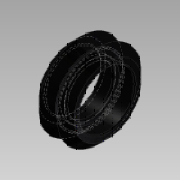
# Autodesk Inventor part: Dual V Wheel
Saved by Autodesk Inventor 2013 SP2 (Build 170200200, 200)
## iProperties
Created: 2013-06-20
Part Number: Dual V Wheel
Material: Acetal Resin, Black
Document SubType Name: Modeling
Designer: Jon Hollander
Language: en-US
Size Designation: Dual V Wheel
Categories: <MemberInstance><Categories><Category DisplayName="Other Parts" InternalName="5aa15e00-363f-49f2-933f-16f664388e3f" Mnemonic="OTHER"><Category DisplayName="Wheel Parts" InternalName="9b824a2a-da77-471e-9ca4-422f1cf2c5b3" Mnemonic="WHEEL PARTS"/></Category><Category DisplayName="DataType" InternalName="23b78d0f-2648-40c6-8793-ca6db495c9e8" Mnemonic="DATATYPE"><CategoryParameter DisplayName="DisplayName" InternalName="05415f3d-3907-474b-a020-eb9d644f4cf3" Mnemonic="DISPLAYNAME"/><CategoryParameter DisplayName="InternalName" InternalName="cf1d0246-76d9-4b4a-8305-fa0409afb5c1" Mnemonic="INTERNALNAME"/><CategoryParameter DisplayName="Folder Name" InternalName="3f06958e-8713-4116-9be7-ed6184ecc97b" Mnemonic="FOLDERNAME"/><CategoryParameter DisplayName="Family Version" InternalName="914462f6-6e19-4b14-ba84-155b9680b1d0" Mnemonic="FAMILYREVISION"/><CategoryParameter DisplayName="ClipFormat" InternalName="bc51e27b-3422-4e78-93ef-cec197ddf230" Mnemonic="CLIPFORMAT"/><CategoryParameter DisplayName="IsMetric" InternalName="e2385c5b-1ea4-4823-96a8-8de651266ec3" Mnemonic="ISMETRIC"/><CategoryParameter DisplayName="Description" InternalName="13903e3d-64b1-4950-80da-f627842ea37f" Mnemonic="DESCRIPTION"/><CategoryParameter DisplayName="StdsOrg" InternalName="8f5914e1-4693-403f-8ab5-d37768198c9d" Mnemonic="STDSORG"/><CategoryParameter DisplayName="Standard" InternalName="0c0a119c-1e12-4c84-803f-101930972f5e" Mnemonic="STANDARD"/><CategoryParameter DisplayName="Manufacturer" InternalName="cd6c7a72-a28a-4e50-99a9-2c7f4e13e5ad" Mnemonic="MANUFACTURER"/><CategoryParameter DisplayName="Member Revision" InternalName="a65d44b9-392f-4f4f-857b-e4b3d54996fe" Mnemonic="MEMBERREVISION"/><CategoryParameter DisplayName="Standard Revision" InternalName="91d5a463-65c2-4fde-b823-3b7fea5e8e17" Mnemonic="STANDARDREVISION"/><CategoryParameter DisplayName="Revision Guid" InternalName="45a75005-10b1-4dfc-8d6d-dfe629f0b93c" Mnemonic="REVISIONGUID"/><CategoryParameter DisplayName="Designation" InternalName="2675968c-4ce5-49e0-a4f5-552d29089031" Mnemonic="DESIGNATION"/><CategoryParameter DisplayName="FileName" InternalName="8b46a4cc-9585-4fed-90c3-899f57e09a73" Mnemonic="FILENAME"/><CategoryParameter DisplayName="Default Row" InternalName="2af9ec52-faaa-4026-b378-f9fa4afca842" Mnemonic="DEFAULTROW"/><Category DisplayName="Part" InternalName="c0e0b642-3bcb-4cc8-9e80-f96d35c4afa4" Mnemonic="PART"><CategoryParameter DisplayName="Material" InternalName="818a152a-d3c3-49ca-80ee-df7d91421b8e" Mnemonic="MATERIAL"/><CategoryParameter DisplayName="Material Key" InternalName="5c9a8adb-dd2b-4535-b97f-0a94a95fe41f" Mnemonic="MATERIALKEY"/><CategoryParameter DisplayName="Part Number" InternalName="016b6077-bfbe-49bd-92c9-d8d59c39c941" Mnemonic="PARTNUMBER"/><CategoryParameter DisplayName="Stock Number" InternalName="4dba7c1c-e26c-444e-836c-b08b433409a8" Mnemonic="STOCKNUMBER"/></Category></Category></Categories><FamilyTemplate Id="Dual V Wheel"><FamilyTemplateParameters><FamilyTemplateParameter ObjectType="kPartComponentDefinitionObject" ValueType="xs:string" Id="11" SubObjectId="Material"/><FamilyTemplateParameter ObjectType="kPropertyObject" ValueType="xs:string" Id="13" ObjectReferenceKey="{32853F0F-3444-11d1-9E93-0060B03C1CA6}" SubObjectId="5"/><FamilyTemplateParameter ObjectType="kPropertyObject" ValueType="xs:string" Id="14" ObjectReferenceKey="{32853F0F-3444-11d1-9E93-0060B03C1CA6}" SubObjectId="52"/></FamilyTemplateParameters></FamilyTemplate><CategoryParameterMap><ParamToTemplateMap><ParamToTemplate CategoryParameter="//CategoryParameter[@InternalName='cf1d0246-76d9-4b4a-8305-fa0409afb5c1']" ConstantValue="8048950d-5559-4bd6-817f-6bbe3ec72d64"/><ParamToTemplate CategoryParameter="//CategoryParameter[@InternalName='45a75005-10b1-4dfc-8d6d-dfe629f0b93c']" ConstantValue="1baaf515-ac98-4229-ad65-f93490cf2c77"/><ParamToTemplate CategoryParameter="//CategoryParameter[@InternalName='3f06958e-8713-4116-9be7-ed6184ecc97b']" ConstantValue="Dual V Wheel"/><ParamToTemplate CategoryParameter="//CategoryParameter[@InternalName='8f5914e1-4693-403f-8ab5-d37768198c9d']" TemplateParameter="5"/><ParamToTemplate CategoryParameter="//CategoryParameter[@InternalName='0c0a119c-1e12-4c84-803f-101930972f5e']" TemplateParameter="6"/><ParamToTemplate CategoryParameter="//CategoryParameter[@InternalName='91d5a463-65c2-4fde-b823-3b7fea5e8e17']" TemplateParameter="7"/><ParamToTemplate CategoryParameter="//CategoryParameter[@InternalName='cd6c7a72-a28a-4e50-99a9-2c7f4e13e5ad']" TemplateParameter="8"/><ParamToTemplate CategoryParameter="//CategoryParameter[@InternalName='13903e3d-64b1-4950-80da-f627842ea37f']" TemplateParameter="10"/><ParamToTemplate CategoryParameter="//CategoryParameter[@InternalName='05415f3d-3907-474b-a020-eb9d644f4cf3']" ConstantValue="Dual V Wheel"/><ParamToTemplate CategoryParameter="//CategoryParameter[@InternalName='914462f6-6e19-4b14-ba84-155b9680b1d0']" ConstantValue="11"/><ParamToTemplate CategoryParameter="//CategoryParameter[@InternalName='bc51e27b-3422-4e78-93ef-cec197ddf230']" ConstantValue="CF_INVENTOR.STDPARTS"/><ParamToTemplate CategoryParameter="//CategoryParameter[@InternalName='e2385c5b-1ea4-4823-96a8-8de651266ec3']" ConstantValue="true"/><ParamToTemplate CategoryParameter="//CategoryParameter[@InternalName='2af9ec52-faaa-4026-b378-f9fa4afca842']" ConstantValue="1"/><ParamToTemplate CategoryParameter="//CategoryParameter[@InternalName='8b46a4cc-9585-4fed-90c3-899f57e09a73']" ConstantValue="Dual V Wheel"/><ParamToTemplate CategoryParameter="//CategoryParameter[@InternalName='a65d44b9-392f-4f4f-857b-e4b3d54996fe']" ConstantValue="3d5e0127-4738-49eb-be70-5cb701e0a2ad"/><ParamToTemplate CategoryParameter="//CategoryParameter[@InternalName='a65d44b9-392f-4f4f-857b-e4b3d54996fe']" ConstantValue="3d5e0127-4738-49eb-be70-5cb701e0a2ad"/><ParamToTemplate CategoryParameter="//CategoryParameter[@InternalName='2675968c-4ce5-49e0-a4f5-552d29089031']" TemplateParameter="14"/><ParamToTemplate CategoryParameter="//CategoryParameter[@InternalName='818a152a-d3c3-49ca-80ee-df7d91421b8e']" TemplateParameter="11"/><ParamToTemplate CategoryParameter="//CategoryParameter[@InternalName='016b6077-bfbe-49bd-92c9-d8d59c39c941']" TemplateParameter="13"/></ParamToTemplateMap></CategoryParameterMap></MemberInstance>
Mass: 2.60986 g
Surface Area: 18.1288 cm^2
Volume: 1.83148 cm^3
Density: 1.425 g/cm^3
IsCustomPart: 0
Author: Jon Hollander
Autodesk Inventor part; units mm, degrees
ref_plane "YZ Plane" through (0, 0, 0) normal (1, 0, 0) x (0, 1, 0)
ref_plane "XZ Plane" through (0, 0, 0) normal (0, 1, 0) x (-1, 0, 0)
ref_plane "XY Plane" through (0, 0, 0) normal (0, 0, 1) x (1, 0, 0)
sketch "Sketch1" plane through (0, 0, 0) normal (0, 0, 1) x (1, 0, 0)
  line L0 (0, 0) -> (10, 0)
  line L1 (0, 0) -> (0, 6.945) construction
  line L2 (0, 6.945) -> (0.5, 6.945)
  line L3 (0.5, 6.945) -> (0.5, 7.987)
  line L4 (0.5, 7.987) -> (4.82, 7.987)
  line L5 (5.12, 8.287) -> (5.12, 9.77)
  line L6 (5.12, 9.77) -> (2.695, 12.195)
  line L7 (2.695, 12.195) -> (0.275, 9.775)
  line L8 (0.275, 9.775) -> (0.275, 9.375)
  line L9 (0.275, 9.375) -> (0, 9.375)
  line L10 (4.82, 7.987) -> (5.12, 8.287)
  line L11 (0, 6.945) -> (0, 11.2763) construction
  line L12 (0, 6.945) -> (-0.5, 6.945)
  line L13 (-0.5, 6.945) -> (-0.5, 7.987)
  line L14 (-0.5, 7.987) -> (-4.82, 7.987)
  line L15 (-5.12, 8.287) -> (-5.12, 9.77)
  line L16 (-5.12, 9.77) -> (-2.695, 12.195)
  line L17 (-2.695, 12.195) -> (-0.275, 9.775)
  line L18 (-0.275, 9.775) -> (-0.275, 9.375)
  line L19 (-0.275, 9.375) -> (0, 9.375)
  line L20 (-4.82, 7.987) -> (-5.12, 8.287)
  point P0 (5.12, 7.987)
  point P1 (-5.12, 7.987)
  dimension "d0" = 10
  dimension "d2" = 0.5
  dimension "d3" = 15.974
  dimension "d4" = 13.89
  dimension "d5" = 0.3
  dimension "d6" = 0.3
  dimension "d7" = 19.54
  dimension "d8" = 5.12
  dimension "d12" = 24.39
  dimension "d14" = 18.75
  dimension "d16" = 0.275
  dimension "d17" = 135
  dimension "d18" = 135
  dimension "d19" = 2.695
  constraints: 42 end point, 9 symmetric about line, 5 point on line, 4 parallel, 4 perpendicular, 1 horizontal
  measures "d0" distance of L0.start L0.end
  measures "d2" distance of L1.end L2.end
  measures "d3" diameter of L4 L0
  measures "d4" diameter of L2 L0
  measures "d5" distance of L4.end point (5.12, 7.987)
  measures "d6" distance of L5.start point (5.12, 7.987)
  measures "d7" diameter of L5.end L0
  measures "d8" distance between parallel lines of L1 L5
  measures "d12" diameter of L6.end L0
  measures "d14" diameter of L9 L0
  measures "d16" distance between parallel lines of L11 L8
  measures "d17" angle of L5 L6
  measures "d18" angle of L7 L8
  measures "d19" distance from line of L11 L6.end
revolve "Revolution1" add sketch "Sketch1" angle 360 about axis through (0, 0, 0) along (1, 0, 0)
equation "\"d6\" = d5"
body "Solid1"
